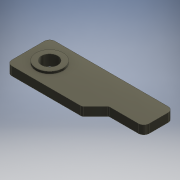
# Autodesk Inventor part: X End Stop Flag 1.0
Saved by Autodesk Inventor 2016 (Build 200138000, 138)
## iProperties
Created: 2017-02-11
Part Number: X End Stop Flag 1.0
Material: PC/ABS Plastic
Document SubType Name: Modeling
Designer: Scott
Density: 0.357273 g/cm^3
Appearance: Gunmetal
Author: Scott
## iProperties of the stored document X End Stop Flag 1.0_3DPrint.ipt
Created: 2017-04-15
Part Number: X End Stop Flag 1.0_3DPrint
Material: Generic
Document SubType Name: Modeling
Designer: Scott
Density: 1 g/cm^3
Appearance: Default
Author: Scott
Autodesk Inventor part; units mm, degrees
ref_plane "YZ Plane" through (0, 0, 0) normal (1, 0, 0) x (0, 1, 0)
ref_plane "XZ Plane" through (0, 0, 0) normal (0, 1, 0) x (-1, 0, 0)
ref_plane "XY Plane" through (0, 0, 0) normal (0, 0, 1) x (1, 0, 0)
sketch "Sketch1" plane through (0, 0, 0) normal (0, 0, 1) x (1, 0, 0)
  circle A0 centre (0, 0) radius 1.5
  line L0 (-4, 4) -> (19, 4)
  line L1 (19, 4) -> (19, -1.5)
  line L2 (10, -4) -> (-4, -4)
  line L3 (-4, -4) -> (-4, 4)
  line L4 (19, -1.5) -> (12.5, -1.5)
  line L5 (10, -4) -> (12.5, -1.5)
  dimension "d0" = 3
  dimension "d1" = 4
  dimension "d2" = 23
  dimension "d3" = 4
  dimension "d4" = 4
  dimension "d6" = 5.5
  dimension "d15" = 14
  dimension "d16" = 135
  constraints: 12 end point, 2 horizontal, 2 parallel, 1 centre point, 1 coincident, 1 perpendicular
  measures "d0" diameter of A0
  measures "d1" distance from line of L3 point (0, 0)
  measures "d2" distance of L0.start L0.end
  measures "d3" distance from line of point (0, 0) L2
  measures "d4" distance from line of point (0, 0) L0
  measures "d6" distance of L0.end L1.end
  measures "d15" distance of L2.start L2.end
  measures "d16" angle of L4 L5
extrude "Extrusion1" add sketch "Sketch1" along normal blind 1.6
sketch "Sketch2" plane through (0, 0, 1.6) normal (0, 0, 1) x (1, 0, 0)
  circle A0 centre (0, 0) radius 1.5 projected
  circle A1 centre (0, 0) radius 1.5
  circle A2 centre (0, 0) radius 2.5
  dimension "d9" = 5
  constraints: 2 centre point, 2 coincident, 1 concentric
  measures "d9" diameter of A2
extrude "Extrusion2" add sketch "Sketch2" along normal blind 0.4
fillet "Fillet1" radius 1 1 edges at (-4, 4, 0.8)
fillet "Fillet2" radius 1 3 edges at (-4, -4, 0.8) (19, -1.5, 0.8) (19, 4, 0.8)
fillet "Fillet3" radius 0.5 2 edges at (10, -4, 0.8) (12.5, -1.5, 0.8)
body "Solid1"
